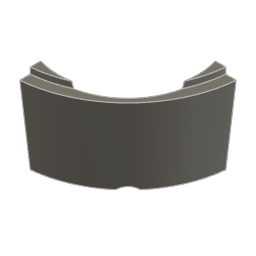
carcasas medias (Autodesk Fusion 360 design; units mm, degrees)
Autodesk Fusion 360 part; units mm, degrees
sketch "Boceto1" plane through (0, 0, 0) normal (0, 0, 1) x (1, 0, 0)
  line L0 (47.5, 0) -> (52.5, 0)
  line L1 (52.5, 40) -> (57.5, 40)
  line L2 (47.5, 40) -> (45, 0)
  line L3 (57.5, 40) -> (52.5, 0)
  line L4 (47.5, 40) -> (47.5, 43)
  line L5 (47.5, 43) -> (52.5, 43)
  line L6 (52.5, 43) -> (52.5, 40)
  line L7 (45, 0) -> (45, -3)
  line L8 (45, -3) -> (47.5, -3)
  line L9 (47.5, -3) -> (47.5, 0)
  dimension "d1" = 45
  dimension "d2" = 7.5
  dimension "d7" = 3
  dimension "d8" = 5
  dimension "d9" = 3
  dimension "d10" = 2.5
  constraint perpendicular L1 L4
  constraint perpendicular L4 L5
  constraint perpendicular L1 L6
  constraint perpendicular L0 L7
  constraint perpendicular L7 L8
  constraint perpendicular L0 L9
  measures "d1" distance of origin L2.end
  measures "d2" distance of L2.end L0.end
  measures "d7" distance of L2.start L4.end
  measures "d8" distance of L4.end L5.end
  measures "d9" distance of L2.end L7.end
  measures "d10" distance of L7.end L8.end
revolve "Revolución1" add sketch "Boceto1" angle 90 about axis through (0, 1.75, 0) along (0, -1, 0)
sketch "Boceto2" plane through (0, 43, 0) normal (0, 1, 0) x (-1, 0, 0)
  line L0 (-52.5, 0) -> (-47.5, 0)
  arc A0 (0, 47.5) -> (-47.5, 0) centre (0, 0) ccw
  line L1 (0, 47.5) -> (0, 52.5)
  arc A1 (0, 52.5) -> (-52.5, 0) centre (0, 0) ccw
  line L2 (-44.5, 0) -> (-44.5, 5)
  line L3 (-44.5, 5) -> (-58, 5)
  line L4 (-58, 5) -> (-58, 0)
  line L5 (-58, 0) -> (-44.5, 0)
  line L6 (0, 44) -> (-5, 44)
  line L7 (-5, 44) -> (-5, 58)
  line L8 (-5, 58) -> (0, 58)
  line L9 (0, 58) -> (0, 44)
  dimension "d12" = 5
  constraint vertical L2
  constraint perpendicular L2 L3
  constraint perpendicular L3 L4
  constraint perpendicular L2 L5
  constraint horizontal L6
  constraint perpendicular L6 L7
  constraint perpendicular L7 L8
  constraint perpendicular L6 L9
  measures "d12" distance of L2.start L2.end
extrude "Extruir1" cut sketch "Boceto2" against normal blind 50 contours L0 A0 A1 L3 L5 | A1 L3 L4 L5 | A0 L2 L3 L5 | A1 L7 L8 L9 | A0 L1 A1 L7 L9 | A0 L6 L7 L9
sketch "Boceto3" plane through (0, 43, 0) normal (0, 1, 0) x (-1, 0, 0)
  line L0 (-5, 47.2361) -> (-5, 52.2614)
  arc A0 (-5, 52.2614) -> (-52.2614, 5) centre (0, 0) ccw
  line L1 (-52.2614, 5) -> (-47.2361, 5)
  arc A1 (-5, 47.2361) -> (-47.2361, 5) centre (0, 0) ccw
  line L2 (-21.754, 42.2258) -> (-23.4766, 46.9585)
  line L3 (0, 0) -> (52.5, 0) construction
  line L4 (-42.2258, 21.754) -> (-46.9585, 23.4766)
  line L5 (0, 0) -> (52.5, 0) construction
  arc A2 (-23.4766, 46.9585) -> (-46.9585, 23.4766) centre (0, 0) ccw
  line L6 (-42.2258, 21.754) -> (-41.2783, 21.4091)
  line L7 (-42.2258, 21.754) -> (-43.6353, 21.754) construction
  line L8 (-21.754, 42.2258) -> (-21.4091, 41.2783)
  arc A3 (-21.4091, 41.2783) -> (-41.2783, 21.4091) centre (0, 0) ccw
  dimension "d15" = 110
  dimension "d16" = 160
  dimension "d17" = 93
  dimension "d18" = 20
  constraint horizontal L3
  constraint coincident A0.centre A1.centre
  constraint horizontal L5
  constraint coincident A1 L4.start
  constraint coincident A1 L2.start
  constraint horizontal L7
  constraint parallel L2 L8
  measures "d15" angle of L2 L3
  measures "d16" angle of L4 L5
  measures "d17" diameter of A3
  measures "d18" angle of L6 L7
extrude "Extruir2" cut sketch "Boceto3" against normal blind 10 contours A1 L6 L8 A3 | A0 A1 L2 L4 A2
sketch "Boceto4" plane through (0, -3, 0) normal (0, -1, 0) x (1, 0, 0)
  line L0 (5, 47.2361) -> (5, 44.7214)
  arc A0 (44.7214, 5) -> (5, 44.7214) centre (0, 0) ccw
  line L1 (44.7214, 5) -> (47.2361, 5)
  arc A1 (47.2361, 5) -> (5, 47.2361) centre (0, 0) ccw
  line L2 (42.2862, 15.3909) -> (44.6354, 16.246)
  line L3 (15.3909, 42.2862) -> (16.246, 44.6354)
  arc A2 (44.6354, 16.246) -> (16.246, 44.6354) centre (0, 0) ccw
  arc A3 (42.2862, 15.3909) -> (15.3909, 42.2862) centre (0, 0) ccw
  constraint coincident A0.centre A1.centre
  constraint coincident A1 L2.end
  constraint coincident A0 L2.start
  constraint coincident A0 L3.start
extrude "Extruir3" cut sketch "Boceto4" against normal blind 10 contours A0 A1 L2 L3 A2 A3
sketch "Boceto5" plane through (0, 40, 0) normal (0, 1, 0) x (-1, 0, 0)
  line L0 (-5, 52.2614) -> (-5, 57.2822)
  arc A0 (-5, 57.2822) -> (-57.2822, 5) centre (0, 0) ccw
  line L1 (-57.2822, 5) -> (-52.2614, 5)
  arc A1 (-46.9585, 23.4766) -> (-52.2614, 5) centre (0, 0) ccw
  arc A2 (-23.4766, 46.9585) -> (-46.9585, 23.4766) centre (0, 0) ccw
  arc A3 (-5, 52.2614) -> (-23.4766, 46.9585) centre (0, 0) ccw
  circle A4 centre (-15, 15) radius 33.5
  dimension "d26" = 67
  measures "d26" diameter of A4
extrude "Extruir4" cut sketch "Boceto5" against normal blind 45 draft -3 contours A1 A2 A3 A4 | A1 A2 A3 A4
extrude "Extruir5" cut sketch "Boceto5" along normal blind 15 draft 3 contours A1 A2 A3 A4 | A1 A2 A3 A4
extrude "Extruir6" cut sketch "Boceto5" against normal blind 45 draft -3 contours A1 A2 A3 A4 | A1 A2 A3 A4
